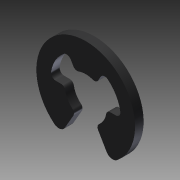
# Autodesk Inventor part: D-5866
Saved by Autodesk Inventor 2011 SP1 (Build 150282100, 282)
## iProperties
Created: 2016-11-12
Part Number: D-5866
Catalog Web Link: www.cadenas.de
Description: Piston Rod Clevis for Original Line Cylinders - Retaining Ring-
Vendor: BIMBA
Document SubType Name: Modeling
Designer: psAdmin
Manufacturer: BIMBA
Mass: 0.0803103 g
Surface Area: 2.14447 cm^2
Volume: 0.0803103 cm^3
Density: 1 g/cm^3
Category: PARTsolutions
Company: BIMBA
Title: D-5866
Author: Cadenas PARTsolutions
PSOL_IDENT_0: {$CADENAS_DATA\23d-libs\bimba\bimba\bimba_imperial\bimba_full_line\original_line_cylinders\accessori
PSOL_IDENT_1: es\piston_rod_clevis_rr.prj},211 {VTYP=3D},{NB=D-5866},{LINA=D-5866},{NN=Piston Rod Clevis for Origi
PSOL_IDENT_2: nal Line Cylinders - Retaining Ring},{DATE=09.11.2016 07:55:10},{GEOMDATE=06.12.2012 07:18:40},{VERS
PSOL_IDENT_3: ION=},{LINEID=190},{LINESUBID=-1},{WBVAR=}  {NB=D-5866},{LINA=D-5866},{KT=DUMMY},{PN=D-5866},{D=0.50
PSOL_IDENT_4: 000000},{D1=0.21050000},{D2=0.35525},{L=0.04350000},{COLOR=0.75,0.75,0.75,0.00}
NN: Piston Rod Clevis for Original Line Cylinders - Retaining Ring
NB: D-5866
NBSYN: $PN.
LINA: D-5866
PN: D-5866
D: 0.50000000
D1: 0.21050000
L: 0.04350000
SUPPLIER: BIMBA
ARTICLENO: D-5866
BOMINFO: D-5866
CREATOR: CADENAS GmbH
Autodesk Inventor part; units mm, degrees
sketch "Sketch_1" plane through (0, 0, 0) normal (0, 0, 1) x (1, 0, 0)
  arc A0 (4.042, -4.8974) -> (-4.042, -4.8974) centre (0, 0) ccw
  arc A1 (-4.042, -4.8974) -> (-2.6862, -4.6526) centre (-3.4677, -4.2015) ccw
  line L0 (-2.6862, -4.6526) -> (-1.5816, -2.7394)
  arc A2 (-1.5816, -2.7394) -> (-1.7038, -2.06) centre (-2.0446, -2.472) ccw
  arc A3 (-2.636, -0.4456) -> (-1.7038, -2.06) centre (0, 0) ccw
  arc A4 (-2.636, -0.4456) -> (-3.1632, 0) centre (-3.1632, -0.5347) ccw
  line L1 (-3.1632, 0) -> (-3.8636, 0)
  arc A5 (-4.458, 0.6941) -> (-3.8636, 0) centre (-3.8636, 0.6016) ccw
  arc A6 (-2.8301, 3.5137) -> (-4.458, 0.6941) centre (0, 0) ccw
  arc A7 (-1.9318, 3.3459) -> (-2.8301, 3.5137) centre (-2.4527, 3.0452) ccw
  line L2 (-1.9318, 3.3459) -> (-1.5816, 2.7394)
  arc A8 (-1.5816, 2.7394) -> (-0.9321, 2.5056) centre (-1.1185, 3.0067) ccw
  arc A9 (0.9321, 2.5056) -> (-0.9321, 2.5056) centre (0, 0) ccw
  arc A10 (0.9321, 2.5056) -> (1.5816, 2.7394) centre (1.1185, 3.0067) ccw
  line L3 (1.5816, 2.7394) -> (1.9318, 3.3459)
  arc A11 (2.8301, 3.5137) -> (1.9318, 3.3459) centre (2.4527, 3.0452) ccw
  arc A12 (4.458, 0.6941) -> (2.8301, 3.5137) centre (0, 0) ccw
  arc A13 (3.8636, 0) -> (4.458, 0.6941) centre (3.8636, 0.6016) ccw
  line L4 (3.8636, 0) -> (3.1632, 0)
  arc A14 (3.1632, 0) -> (2.636, -0.4456) centre (3.1632, -0.5347) ccw
  arc A15 (1.7038, -2.06) -> (2.636, -0.4456) centre (0, 0) ccw
  arc A16 (1.7038, -2.06) -> (1.5816, -2.7394) centre (2.0446, -2.472) ccw
  line L5 (1.5816, -2.7394) -> (2.6862, -4.6526)
  arc A17 (2.6862, -4.6526) -> (4.042, -4.8974) centre (3.4677, -4.2015) ccw
  constraints: 36 point on circle, 18 centre point, 12 end point
extrude "Extrusion1" add sketch "Sketch_1" along normal mid plane 1.1049
ref_plane "RR_XY" through (0, 0, 0) normal (0, 0, 1) x (1, 0, 0)
ref_plane "RR_YZ" through (0, 0, 0) normal (1, 0, 0) x (0, 1, 0)
ref_plane "RR_ZX" through (0, 0, 0) normal (0, 1, 0) x (0, 0, 1)
body "Solid1"
